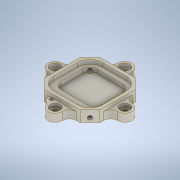
# Autodesk Inventor part: 로드셀 케이스2
Saved by Autodesk Inventor 2021 (Build 250183000, 183)
## iProperties
Created: 2021-08-10
Part Number: 로드셀 케이스2
Material: 티타늄
Document SubType Name: Modeling
Designer: Dongyoon
Density: 4.51 g/cm^3
Appearance: 티타늄
Author: Dongyoon
Autodesk Inventor part; units mm, degrees
ref_plane "YZ Plane" through (0, 0, 0) normal (1, 0, 0) x (0, 1, 0)
ref_plane "XZ Plane" through (0, 0, 0) normal (0, 1, 0) x (-1, 0, 0)
sketch "스케치1" plane through (0, 0, 0) normal (0, 1, 0) x (-1, 0, 0)
  line L0 (19.5, -19.5) -> (-19.5, -19.5)
  line L1 (-19.5, -19.5) -> (-19.5, 19.5)
  line L2 (-19.5, 19.5) -> (19.5, 19.5)
  line L3 (19.5, 19.5) -> (19.5, -19.5)
  line L4 (19.5, -19.5) -> (-19.5, 19.5) construction
  line L5 (-19.5, -19.5) -> (19.5, 19.5) construction
  point P0 (0, 0)
  dimension "d0" = 39
  dimension "d1" = 39
  constraints: 12 end point, 2 midpoint, 2 parallel, 1 horizontal, 1 perpendicular
  measures "d0" distance of L1.end L2.end
  measures "d1" distance of L0.end L1.end
extrude "돌출1" add sketch "스케치1" along normal blind 5
sketch "스케치2" plane through (0, 5, 0) normal (0, 1, 0) x (1, 0, 0)
  line L0 (-19.5, -19.5) -> (19.5, -19.5) projected
  line L1 (-19.5, 19.5) -> (19.5, 19.5)
  line L2 (19.5, 19.5) -> (19.5, -19.5)
  line L3 (19.5, -19.5) -> (-19.5, -19.5)
  line L4 (-19.5, -19.5) -> (-19.5, 19.5)
  line L5 (-19.5, 19.5) -> (19.5, -19.5) construction
  line L6 (19.5, 19.5) -> (-19.5, -19.5) construction
  line L7 (-8.25, 17.25) -> (8.25, 17.25)
  line L8 (17.25, 8.25) -> (17.25, -8.25)
  line L9 (8.25, -17.25) -> (-8.25, -17.25)
  line L10 (-17.25, -8.25) -> (-17.25, 8.25)
  line L11 (-17.25, 17.25) -> (17.25, -17.25) construction
  line L12 (17.25, 17.25) -> (-17.25, -17.25) construction
  arc A0 (-8.25, 17.25) -> (-17.25, 8.25) centre (-8.25, 8.25) ccw
  arc A1 (17.25, 8.25) -> (8.25, 17.25) centre (8.25, 8.25) ccw
  arc A2 (8.25, -17.25) -> (17.25, -8.25) centre (8.25, -8.25) ccw
  arc A3 (-17.25, -8.25) -> (-8.25, -17.25) centre (-8.25, -8.25) ccw
  point P0 (0, 0)
  dimension "d4" = 34.5
  dimension "d5" = 9
  constraints: 24 end point, 9 point on line, 8 point on circle, 8 tangent, 4 centre point, 4 midpoint, 4 parallel, 3 equal radius, 2 horizontal, 2 perpendicular
  measures "d4" distance of L12.start L11.end
  measures "d5" radius of A0
extrude "돌출2" add sketch "스케치2" along normal blind 2.7
sketch "스케치3" plane through (0, 5, 0) normal (0, 1, 0) x (1, 0, 0)
  line L0 (-14.25, 9.25) -> (-14.25, -6.25)
  line L1 (-9.25, -11.25) -> (9.25, -11.25)
  line L2 (14.25, -6.25) -> (14.25, 9.25)
  line L3 (9.25, 14.25) -> (-9.25, 14.25)
  line L4 (-8.25, 17.25) -> (8.25, 17.25) projected
  line L5 (-17.25, -8.25) -> (-17.25, 8.25) projected
  line L6 (17.25, 8.25) -> (17.25, -8.25) projected
  line L7 (8.25, -17.25) -> (-8.25, -17.25) projected
  arc A0 (-9.25, 14.25) -> (-14.25, 9.25) centre (-9.25, 9.25) ccw
  arc A1 (14.25, 9.25) -> (9.25, 14.25) centre (9.25, 9.25) ccw
  arc A2 (9.25, -11.25) -> (14.25, -6.25) centre (9.25, -6.25) ccw
  arc A3 (-14.25, -6.25) -> (-9.25, -11.25) centre (-9.25, -6.25) ccw
  point P0 (0, 0)
  dimension "d8" = 3
  dimension "d9" = 3
  dimension "d10" = 3
  dimension "d11" = 6
  dimension "d12" = 5
  constraints: 8 end point, 8 point on circle, 8 tangent, 4 centre point, 3 equal radius, 3 perpendicular, 1 vertical
  measures "d8" distance between parallel lines of L4 L3
  measures "d9" distance between parallel lines of L5 L0
  measures "d10" distance between parallel lines of L6 L2
  measures "d11" distance between parallel lines of L7 L1
  measures "d12" radius of A0
extrude "돌출3" cut sketch "스케치3" against normal blind 3
sketch "스케치4" plane through (0, 0, 0) normal (0, 1, 0) x (-1, 0, 0)
  line L0 (-19.5, -19.5) -> (19.5, -19.5) projected
  line L1 (5, -29.5) -> (-5, -29.5)
  line L2 (-5, -29.5) -> (-5, -19.5)
  line L3 (-5, -19.5) -> (5, -19.5)
  line L4 (5, -19.5) -> (5, -29.5)
  line L5 (5, -29.5) -> (-5, -19.5) construction
  line L6 (-5, -29.5) -> (5, -19.5) construction
  line L7 (-19.5, 19.5) -> (-19.5, -19.5) projected
  line L8 (-29.5, -5) -> (-19.5, -5)
  line L9 (-19.5, -5) -> (-19.5, 5)
  line L10 (-19.5, 5) -> (-29.5, 5)
  line L11 (-29.5, 5) -> (-29.5, -5)
  line L12 (-29.5, -5) -> (-19.5, 5) construction
  line L13 (-19.5, -5) -> (-29.5, 5) construction
  line L14 (19.5, -19.5) -> (19.5, 19.5) projected
  line L15 (29.5, 5) -> (19.5, 5)
  line L16 (19.5, 5) -> (19.5, -5)
  line L17 (19.5, -5) -> (29.5, -5)
  line L18 (29.5, -5) -> (29.5, 5)
  line L19 (29.5, 5) -> (19.5, -5) construction
  line L20 (19.5, 5) -> (29.5, -5) construction
  line L21 (19.5, 19.5) -> (-19.5, 19.5) projected
  line L22 (5, 19.5) -> (-5, 19.5)
  line L23 (-5, 19.5) -> (-5, 29.5)
  line L24 (-5, 29.5) -> (5, 29.5)
  line L25 (5, 29.5) -> (5, 19.5)
  line L26 (5, 19.5) -> (-5, 29.5) construction
  line L27 (5, 29.5) -> (-5, 19.5) construction
  point P0 (0, 0)
  point P1 (0, -24.5)
  point P2 (-24.5, 0)
  point P3 (24.5, 0)
  point P4 (0, 24.5)
  dimension "d15" = 10
  dimension "d16" = 10
  dimension "d18" = 10
  dimension "d19" = 10
  dimension "d20" = 5
  dimension "d21" = 10
  dimension "d22" = 5
  dimension "d23" = 10
  dimension "d24" = 10
  dimension "d25" = 10
  dimension "d26" = 5
  constraints: 48 end point, 8 parallel, 7 midpoint, 5 point on line, 4 horizontal, 4 perpendicular
  measures "d15" distance of L1.start L1.end
  measures "d16" distance of L10.end L8.start
  measures "d18" distance of L17.end L15.start
  measures "d19" distance of L16.end L17.end
  measures "d20" distance from line of point (0, 0) L17
  measures "d21" distance of L1.end L2.end
  measures "d22" distance from line of L4 point (0, 0)
  measures "d23" distance of L8.start L8.end
  measures "d24" distance of L22.end L23.end
  measures "d25" distance of L23.end L24.end
  measures "d26" distance from line of point (0, 0) L23
extrude "돌출4" add sketch "스케치4" along normal blind 5.5 contours L0 L4 L1 L2 | L8 L11 L10 L7 | L14 L15 L18 L17 | L23 L24 L25 L21
sketch "스케치5" plane through (0, 5.5, 0) normal (0, 1, 0) x (1, 0, 0)
  circle A0 centre (-24.5, 0) radius 1.95
  line L0 (-19.5, 19.5) -> (-19.5, -19.5) projected
  line L1 (-29.5, -5) -> (-19.5, -5) projected
  circle A1 centre (0, 24.5) radius 1.95
  line L2 (5, 19.5) -> (5, 29.5) projected
  line L3 (19.5, 19.5) -> (-19.5, 19.5) projected
  circle A2 centre (24.5, 0) radius 1.95
  line L4 (29.5, -5) -> (29.5, 5) projected
  line L5 (19.5, -5) -> (29.5, -5) projected
  circle A3 centre (0, -24.5) radius 1.95
  line L6 (5, -29.5) -> (5, -19.5) projected
  line L7 (-5, -29.5) -> (5, -29.5) projected
  dimension "d29" = 3.9
  dimension "d30" = 5
  dimension "d31" = 5
  dimension "d32" = 3.9
  dimension "d33" = 5
  dimension "d34" = 5
  dimension "d35" = 3.9
  dimension "d36" = 5
  dimension "d37" = 5
  dimension "d38" = 3.9
  dimension "d39" = 5
  dimension "d40" = 5
  constraints: 4 centre point
  measures "d29" diameter of A0
  measures "d30" distance from line of L0 A0.centre
  measures "d31" distance from line of L1 A0.centre
  measures "d32" diameter of A1
  measures "d33" distance from line of L2 A1.centre
  measures "d34" distance from line of L3 A1.centre
  measures "d35" diameter of A2
  measures "d36" distance from line of L4 A2.centre
  measures "d37" distance from line of L5 A2.centre
  measures "d38" diameter of A3
  measures "d39" distance from line of L6 A3.centre
  measures "d40" distance from line of L7 A3.centre
extrude "돌출5" cut sketch "스케치5" against normal through all
sketch "스케치6" plane through (0, 5.5, 0) normal (0, 1, 0) x (1, 0, 0)
  circle A0 centre (-24.5, 0) radius 1.95 projected
  circle A1 centre (-24.5, 0) radius 3.5
  circle A2 centre (0, 24.5) radius 1.95 projected
  circle A3 centre (0, 24.5) radius 3.5
  circle A4 centre (24.5, 0) radius 1.95 projected
  circle A5 centre (24.5, 0) radius 3.5
  circle A6 centre (0, -24.5) radius 1.95 projected
  circle A7 centre (0, -24.5) radius 3.5
  point P0 (0, 0)
  dimension "d43" = 7
  dimension "d44" = 7
  dimension "d45" = 7
  dimension "d46" = 7
  constraints: 4 centre point, 4 coincident
  measures "d43" diameter of A7
  measures "d44" diameter of A5
  measures "d45" diameter of A3
  measures "d46" diameter of A1
extrude "돌출6" cut sketch "스케치6" against normal blind 2.5 contours A0 | A1 | A3 | A4 | A5 | A7
fillet "모깎기1" radius 5 8 edges at (5, 2.75, 29.5) (-5, 2.75, 29.5) (29.5, 2.75, -5) (29.5, 2.75, 5) (-5, 2.75, -29.5) (5, 2.75, -29.5) (-29.5, 2.75, 5) (-29.5, 2.75, -5)
fillet "모깎기3" radius 5 7 edges at (19.5, 2.75, -5) (5, 2.75, -19.5) (-5, 2.75, -19.5) (-19.5, 2.75, -5) (-19.5, 2.75, 5) (5, 2.75, 19.5) (19.5, 2.75, 5)
chamfer "모따기1" distance 7 angle 45 4 edges at (-19.5, 3.85, -19.5) (-19.5, 3.85, 19.5) (19.5, 3.85, 19.5) (19.5, 3.85, -19.5)
sketch "스케치8" plane through (12.5, 0, 19.5) normal (0.7071068, 0, 0.7071068) x (0.7071068, 0, -0.7071068)
  circle A0 centre (4.9497, 3) radius 1.4
  line L0 (0, 0) -> (9.8995, 0) projected
  line L1 (9.8995, 0) -> (9.8995, 7.7) projected
  line L2 (9.8995, 7.7) -> (0, 7.7) projected
  line L3 (4.9497, 7.7) -> (4.9497, -2.2168)
  point P0 (4.9497, 0)
  dimension "d59" = 2.8
  dimension "d60" = 3
  constraints: 2 end point, 1 centre point, 1 midpoint, 1 point on line, 1 vertical
  measures "d59" diameter of A0
  measures "d60" distance from line of L0 A0.centre
extrude "돌출7" cut sketch "스케치8" against normal blind 6 contours A0 L3 | L3 A0
ref_plane "작업 평면1" through (-3.5, 0, 3.5) normal (0.7071068, 0, 0.7071068) x (0.7071068, 0, -0.7071068)
mirror "미러1" about plane through (-3.5, 0, 3.5) normal (0.7071068, 0, 0.7071068) of "돌출7"
mirror "미러2" about plane through (0, 0, 0) normal (1, 0, 0) of "돌출7", "미러1"
sketch "스케치15" plane through (0, 5.5, 0) normal (0, 1, 0) x (1, 0, 0)
  line L0 (-12.5, -19.5) -> (-5, -19.5) projected
  line L1 (-5, -19.5) -> (-9, -19.5)
  line L2 (-9, -19.5) -> (-9, -23.5)
  line L3 (-9, -23.5) -> (-5, -23.5)
  line L4 (-5, -23.5) -> (-5, -19.5)
  circle A0 centre (-6.2, -20.7) radius 1.2
  point P0 (0, 0)
  point P1 (-5, -20.7)
  point P2 (-6.2, -19.5)
  dimension "d100" = 4
  dimension "d101" = 4
  dimension "d102" = 2.4
  constraints: 8 end point, 2 parallel, 2 tangent, 1 centre point, 1 horizontal, 1 perpendicular
  measures "d100" distance of L1.end L2.end
  measures "d101" distance of L2.end L3.end
  measures "d102" diameter of A0
extrude "돌출12" add sketch "스케치15" against normal blind 3 contours L0 A0 L4 L3 L2 | L0 L4 A0
fillet "모깎기5" radius 5 2 edges at (-5, 4, 23.5) (-9, 4, 23.5)
